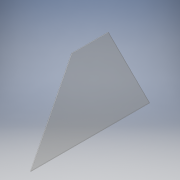
# Autodesk Inventor part: Polycarb Side1 Pannel
Saved by Autodesk Inventor 2016 (Build 200138000, 138)
## iProperties
Created: 2018-05-16
Part Number: Polycarb Side1 Pannel
Material: Polycarbonate, Clear
Document SubType Name: Modeling
Designer: Kade
Density: 1.2 g/cm^3
Appearance: Polycarbonate - Clear
Mass: 1475.73 g
Surface Area: 7834.71 cm^2
Volume: 1229.78 cm^3
Author: Kade
Autodesk Inventor part; units mm, degrees
ref_plane "YZ Plane" through (0, 0, 0) normal (1, 0, 0) x (0, 1, 0)
ref_plane "XZ Plane" through (0, 0, 0) normal (0, 1, 0) x (-1, 0, 0)
ref_plane "XY Plane" through (0, 0, 0) normal (0, 0, 1) x (1, 0, 0)
sketch "Sketch1" plane through (0, 0, 0) normal (1, 0, 0) x (0, 1, 0)
  line L0 (0, 0) -> (0, 660.4)
  line L1 (0, 330.2) -> (453.6585, 330.2) construction
  line L2 (453.6585, 431.8) -> (453.6585, 330.2)
  line L3 (453.6585, 330.2) -> (453.6585, 228.6)
  line L4 (453.6585, 431.8) -> (0, 660.4)
  line L5 (453.6585, 228.6) -> (0, 0)
  dimension "d0" = 660.4
  dimension "d4" = 203.2
  dimension "d29" = 228.6
  dimension "d31" = 508
  dimension "d32" = 453.6585
  constraints: 12 end point, 2 vertical, 1 horizontal, 1 midpoint, 1 parallel
  measures "d0" distance of L0.start L0.end
  measures "d4" distance of L3.end L2.start
  measures "d29" vertical distance of L0.end L2.start
  measures "d31" distance of L3.end L0.start
  measures "d32" distance between parallel lines of L0 L2
extrude "Extrusion1" add sketch "Sketch1" along normal blind 3.175
body "Solid1"
